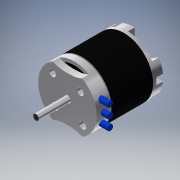
# Autodesk Inventor part: Motor
Saved by Autodesk Inventor 2016 (Build 200138000, 138)
## iProperties
Created: 2015-09-20
Part Number: Motor
Material: Steel
Document SubType Name: Modeling
Designer: Artur
Density: 7.85 g/cm^3
Appearance: Plate
Mass: 50.7671 g
Surface Area: 68.5057 cm^2
Volume: 6.46715 cm^3
Author: Artur
Autodesk Inventor part; units mm, degrees
sketch "Sketch1" plane through (0, 0, 0) normal (0, 1, 0) x (-1, 0, 0)
  circle A0 centre (0, 0) radius 13
  dimension "d0" = 26
  constraints: 1 centre point, 1 coincident
  measures "d0" diameter of A0
extrude "Extrusion1" add sketch "Sketch1" along normal blind 18.5
sketch "Sketch2" plane through (0, 18.5, 0) normal (0, 1, 0) x (1, 0, 0)
  circle A0 centre (0, 0) radius 13 projected
extrude "Extrusion2" add sketch "Sketch2" along normal blind 1.5 separate body
sketch "Sketch3" plane through (0, 20, 0) normal (0, 1, 0) x (1, 0, 0)
  circle A0 centre (0, 0) radius 10.5
  dimension "d5" = 21
  constraints: 1 centre point, 1 coincident
  measures "d5" diameter of A0
extrude "Extrusion3" cut sketch "Sketch3" against normal up to surface (20 mm away) from surface at 0 bodies 2
sketch "Sketch4" plane through (0, 0, 0) normal (0, -1, 0) x (1, 0, 0)
  circle A0 centre (0, 0) radius 10.5
  dimension "d8" = 21
  constraints: 1 centre point, 1 coincident
  measures "d8" diameter of A0
extrude "Extrusion4" cut sketch "Sketch4" against normal up to next bodies 1
ref_plane "Work Plane1" through (0, 20, 0) normal (0, 1, 0) x (1, 0, 0)
sketch "Sketch5" plane through (0, 20, 0) normal (0, 1, 0) x (1, 0, 0)
  circle A0 centre (0, 0) radius 4
  dimension "d12" = 8
  constraints: 1 centre point, 1 coincident
  measures "d12" diameter of A0
extrude "Extrusion5" add sketch "Sketch5" along normal blind 4.5 bodies 2
sketch "Sketch6" plane through (0, 20, 0) normal (0, 1, 0) x (1, 0, 0)
  circle A0 centre (0, 0) radius 4 projected
  circle A1 centre (0, 0) radius 13 projected
  circle A2 centre (6.25, 0) radius 1.25
  circle A3 centre (0, 0) radius 13 projected
  line L0 (-18.3175, 0) -> (18.9053, 0) projected
  circle A4 centre (0, 0) radius 4 projected
  arc A5 (11.0694, -6.8168) -> (12.9132, -1.5) centre (0, 0) ccw
  line L1 (0, 0) -> (12.9132, -1.5) construction
  line L2 (0, 0) -> (11.0694, -6.8168) construction
  line L3 (11.0694, -6.8168) -> (3.406, -2.0975)
  line L4 (12.9132, -1.5) -> (10.9132, -1.5)
  arc A6 (9.4132, 0) -> (10.9132, -1.5) centre (10.9132, 0) ccw
  line L5 (10.9132, 0) -> (9.4132, 0) construction
  line L6 (10.9132, 0) -> (10.9132, -1.5) construction
  arc A7 (12.9132, 1.5) -> (11.0694, 6.8168) centre (0, 0) ccw
  line L7 (11.0694, 6.8168) -> (3.406, 2.0975)
  line L8 (12.9132, 1.5) -> (10.9132, 1.5)
  arc A8 (10.9132, 1.5) -> (9.4132, 0) centre (10.9132, 0) ccw
  arc A9 (3.406, -2.0975) -> (3.406, 2.0975) centre (0, 0) ccw
  dimension "d15" = 2.5
  dimension "d16" = 6.25
  dimension "d19" = 25
  dimension "d20" = 2
  dimension "d21" = 1.5
  dimension "d22" = 90
  constraints: 16 end point, 10 point on circle, 6 centre point, 4 point on line, 4 symmetric about line, 2 coincident, 1 horizontal, 8 other
  measures "d15" diameter of A2
  measures "d16" distance of A2.centre point (0, 0)
  measures "d19" angle of L2 L1
  measures "d20" distance of L1.end L4.end
  measures "d21" distance between parallel lines of L0 L4
  measures "d22" angle of L5 L6
extrude "Extrusion6" add sketch "Sketch6" along normal blind 3 contours L0 A2 A6 L4 A1 L3 A0 | A0 L7 A1 L8 A8 L0 A2 bodies 2
pattern_circular "Circular Pattern1" count 3 over 360 about axis through (0, -10, 0) along (0, 1, 0) of "Extrusion6" bodies 2
sketch "Sketch7" plane through (0, 24.5, 0) normal (0, 1, 0) x (1, 0, 0)
  circle A0 centre (0, 0) radius 1.25
  dimension "d28" = 2.5
  constraints: 1 centre point, 1 coincident
  measures "d28" diameter of A0
extrude "Extrusion7" cut sketch "Sketch7" against normal up to next bodies 2
ref_plane "Work Plane2" through (0, 24.5, 0) normal (0, 1, 0) x (1, 0, 0)
sketch "Sketch8" plane through (0, 24.5, 0) normal (0, 1, 0) x (1, 0, 0)
  circle A0 centre (0, 0) radius 1.25
  dimension "d32" = 2.5
  constraints: 1 centre point, 1 coincident
  measures "d32" diameter of A0
extrude "Extrusion8" add sketch "Sketch8" against normal blind 45 separate body
ref_plane "Work Plane3" through (0, -0.5, 0) normal (0, -1, 0) x (1, 0, 0)
sketch "Sketch9" plane through (0, -0.5, 0) normal (0, -1, 0) x (1, 0, 0)
  circle A0 centre (0, 0) radius 1.25 projected
  circle A1 centre (0, 0) radius 13
  circle A2 centre (0, 0) radius 11.5
  dimension "d36" = 26
  dimension "d37" = 23
  constraints: 2 centre point, 2 coincident
  measures "d36" diameter of A1
  measures "d37" diameter of A2
extrude "Extrusion9" add sketch "Sketch9" along normal blind 3 separate body contours A1
sketch "Sketch10" plane through (0, -3.5, 0) normal (0, -1, 0) x (1, 0, 0)
  circle A0 centre (0, 0) radius 13 construction
  circle A1 centre (0, 0) radius 13 projected
  arc A2 (6.5, -11.2583) -> (13, 0) centre (0, 0) ccw
  line L0 (0, 0) -> (6.5, -11.2583) construction
  line L1 (0, 0) -> (13, 0) construction
  line L2 (0, 0) -> (0, -15.7128) construction
  line L3 (6.5, -11.2583) -> (4.5, -10.1036) construction
  line L4 (4.5, -10.1036) -> (1.75, -10) construction
  line L5 (1.75, -10) -> (0, -10) construction
  spline S0 degree 3 poles (6.5, -11.2583) (4.5, -10.1036) (1.75, -10) (0, -10) knots 1 1 1 1 2 2 2 2
  circle A3 centre (0, 0) radius 13 construction
  line L6 (-6.5, -11.2583) -> (-4.5, -10.1036) construction
  line L7 (-4.5, -10.1036) -> (-1.75, -10) construction
  line L8 (-1.75, -10) -> (0, -10) construction
  spline S1 degree 3 poles (-6.5, -11.2583) (-4.5, -10.1036) (-1.75, -10) (0, -10) knots 1 1 1 1 2 2 2 2
  arc A4 (-13, 0) -> (-6.5, -11.2583) centre (0, 0) ccw
  spline S2 degree 3 poles (-6.5, 11.2583) (-4.5, 10.1036) (-1.75, 10) (0, 10) knots 1 1 1 1 2 2 2 2
  line L9 (-6.5, 11.2583) -> (-4.5, 10.1036) construction
  line L10 (-4.5, 10.1036) -> (-1.75, 10) construction
  line L11 (-1.75, 10) -> (0, 10) construction
  arc A5 (-6.5, 11.2583) -> (-13, 0) centre (0, 0) ccw
  arc A6 (13, 0) -> (6.5, 11.2583) centre (0, 0) ccw
  line L12 (6.5, 11.2583) -> (4.5, 10.1036) construction
  line L13 (4.5, 10.1036) -> (1.75, 10) construction
  line L14 (1.75, 10) -> (0, 10) construction
  spline S3 degree 3 poles (6.5, 11.2583) (4.5, 10.1036) (1.75, 10) (0, 10) knots 1 1 1 1 2 2 2 2
  circle A7 centre (0, 0) radius 1.5
  dimension "d40" = 60
  dimension "d41" = 10
  dimension "d42" = 1.75
  dimension "d43" = 30
  dimension "d44" = 2
  dimension "d47" = 3
  constraints: 11 symmetric about line, 8 point on circle, 6 centre point, 6 end point, 2 coincident, 2 horizontal, 2 horizontal alignment, 1 line through centre, 1 point on line, 1 vertical, 17 other
  measures "d40" angle of L0 L1
  measures "d41" distance of point (0, 0) L5.end
  measures "d42" distance of L5.end L4.end
  measures "d43" angle of L0 L3
  measures "d44" horizontal distance of L0.end L3.end
  measures "d47" diameter of A7
extrude "Extrusion11" add sketch "Sketch10" along normal blind 3 contours A1 S0 S1 S2 S3 bodies 4
sketch "Sketch11" plane through (0, -6.5, 0) normal (0, -1, 0) x (1, 0, 0)
  line L0 (-7.7713, -7.7713) -> (12.2814, 12.2814) construction
  line L1 (-12.926, 12.926) -> (15.5349, -15.5349) construction
  circle A0 centre (-6.7175, 6.7175) radius 1.5
  line L2 (-18.707, 0) -> (21.2418, 0) projected
  line L3 (0, -21.2418) -> (0, 18.707) projected
  circle A1 centre (5.6569, 5.6569) radius 1.5
  circle A2 centre (6.7175, -6.7175) radius 1.5
  circle A3 centre (-5.6569, -5.6569) radius 1.5
  point P0 (0, 0)
  dimension "d50" = 3
  dimension "d51" = 9.5
  dimension "d52" = 45
  dimension "d54" = 3
  dimension "d55" = 8
  constraints: 4 centre point, 4 end point, 4 point on line, 2 symmetric about line, 1 perpendicular, 2 other
  measures "d50" diameter of A0
  measures "d51" distance of point (0, 0) A0.centre
  measures "d52" angle of L0 L2
  measures "d54" diameter of A1
  measures "d55" distance from line of L1 A1.centre
extrude "Extrusion12" cut sketch "Sketch11" against normal up to next bodies 4
ref_plane "Work Plane4" through (13, -6.5, 0) normal (1, 0, 0) x (0, 1, 0)
sketch "Sketch12" plane through (13, -6.5, 0) normal (1, 0, 0) x (0, 1, 0)
  circle A0 centre (3, 4.5) radius 1.25
  line L0 (6, -13) -> (6, 13) projected
  line L1 (-23, 0) -> (40, 0) construction
  circle A1 centre (3, 0) radius 1.25
  circle A2 centre (3, -4.5) radius 1.25
  point P0 (6.5, 0)
  dimension "d58" = 2.5
  dimension "d59" = 3
  dimension "d60" = 4.5
  dimension "d61" = 2.5
  dimension "d62" = 3
  constraints: 3 centre point, 1 point on line, 1 symmetric about line, 1 other
  measures "d58" diameter of A0
  measures "d59" distance from line of L0 A0.centre
  measures "d60" distance from line of L1 A0.centre
  measures "d61" diameter of A1
  measures "d62" distance from line of L0 A1.centre
extrude "Extrusion13" add sketch "Sketch12" against normal up to next separate body
sketch "Sketch13" plane through (13, -3.5, 4.5) normal (1, 0, 0) x (0, 0, -1)
  circle A0 centre (9, 0) radius 1.25 projected
  arc A1 (4.5, 1.25) -> (4.5, -1.25) centre (4.5, 0) ccw projected
  arc A2 (4.5, -1.25) -> (4.5, 1.25) centre (4.5, 0) ccw projected
  circle A3 centre (0, 0) radius 1.25 projected
  point P0 (4.5, 3.5)
extrude "Extrusion14" add sketch "Sketch13" along normal blind 3 bodies 5
